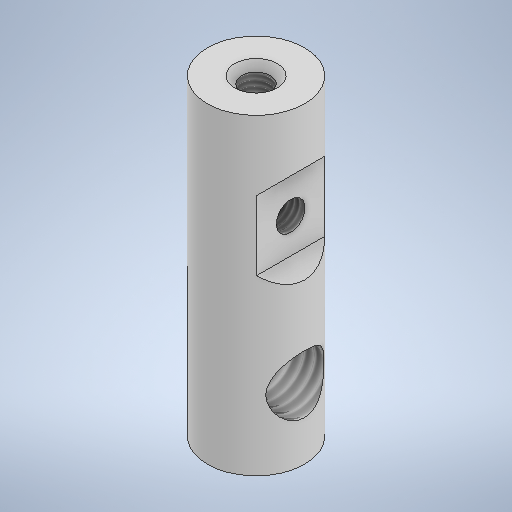
# Autodesk Inventor part: TS_V1_Fallmagazin_Zylinderanbindung_int
Saved by Autodesk Inventor 2025.2 (Build 292293000, 293)
## iProperties
Created: 2025-06-13
Part Number: TS_V1_Fallmagazin_Zylinderanbindung_int
Material: Generisch
Document SubType Name: Modeling
Designer: tino
Density: 1 g/cm^3
Appearance: Vorgabe
Author: tino
Autodesk Inventor part; units mm, degrees
ref_plane "XY Plane" through (0, 0, 0) normal (0, 0, 1) x (1, 0, 0)
sketch "Skizze1" plane through (0, 0, 0) normal (0, 0, 1) x (1, 0, 0)
  circle A0 centre (0, 0) radius 7
  dimension "d0" = 14
  constraints: 1 centre point, 1 coincident
  measures "d0" diameter of A0
extrude "Extrusion1" add sketch "Skizze1" along normal blind 45
sketch "Skizze2" plane through (0, 0, 45) normal (0, 0, 1) x (1, 0, 0)
  circle A0 centre (0, 0) radius 7 projected
hole "Bohrung1" at (0, 0, 45) direction (0, 0, -1) diameter 4.134 depth 11.5 tip angle 118 thread size "M5x0.8" class "6H" standard "ISO Metric profile"
chamfer "Fasen1" distance 1 angle 45 1 edges at (0, 2.067, 45)
ref_plane "Arbeitsebene1" through (-7, 0, 0) normal (1, 0, 0) x (0, 1, 0)
ref_plane "Arbeitsebene2" through (0, -7, 0) normal (0, 1, 0) x (-1, 0, 0)
ref_plane "Arbeitsebene3" through (7, 0, 0) normal (1, 0, 0) x (0, 1, 0)
sketch "Skizze6" plane through (7, 0, 0) normal (1, 0, 0) x (0, 1, 0)
  line L0 (-7, 0) -> (-7, 45) projected
  line L1 (7, 0) -> (7, 45) projected
  line L2 (-7, 25) -> (7, 25)
  line L3 (7, 25) -> (7, 35)
  line L4 (7, 35) -> (-7, 35)
  line L5 (-7, 35) -> (-7, 25)
  line L6 (7, 45) -> (-7, 45) projected
  point P0 (0, 0)
  point P1 (-7, 35)
  dimension "d29" = 10
  dimension "d30" = 10
  constraints: 8 end point, 2 parallel, 2 point on line, 1 horizontal, 1 perpendicular
  measures "d29" distance of L3.end L2.end
  measures "d30" distance between parallel lines of L6 L4
extrude "Extrusion4" cut sketch "Skizze6" against normal blind 2 contours L0 L4 L1 L2
sketch "Skizze7" plane through (5, 0, 0) normal (1, 0, 0) x (0, 0, -1)
  line L0 (-25, -4.899) -> (-25, 4.899) projected
  line L1 (0, 7) -> (0, -7) projected
  point P0 (0, 0)
  point P1 (-30, 0)
  point P2 (0, 0)
  point P3 (0, 0)
  point P4 (0, 0)
  dimension "d33" = 5
  constraints: 1 horizontal alignment, 1 midpoint
  measures "d33" distance from line of point (-30, 0) L0
hole "Bohrung3" at (5, 0, 30) direction (-1, 0, 0) diameter 4.134 end through all thread size "M5x0.8" class "6H" standard "ISO Metric profile"
ref_plane "Arbeitsebene4" through (0, 7, 0) normal (0, 1, 0) x (-1, 0, 0)
sketch "Skizze8" plane through (0, 7, 0) normal (0, 1, 0) x (-1, 0, 0)
  line L0 (-5, 25) -> (-5, 25) projected
  line L1 (-5, 27.933) -> (-5, 32.067) projected
  line L2 (-5, 25) -> (-5, 35) projected
  line L3 (-5, 35) -> (-5, 25) projected
  line L4 (-5, 35) -> (-7, 35) projected
  line L5 (-5, 35) -> (-5, 25) projected
  line L6 (-5, 25) -> (-5, 35) projected
  line L7 (-5, 35) -> (-5, 35) projected
  line L8 (-7, 25) -> (-5, 25) projected
  line L9 (-5, 25) -> (-7, 23)
  line L10 (-7, 0) -> (-7, 45) projected
  line L11 (-5, 25) -> (-2.1716, 25) construction
  line L12 (-7, 23) -> (-7, 25)
  line L13 (-5, 35) -> (-7, 37)
  line L14 (-5, 35) -> (-2.1716, 35) construction
  line L15 (-7, 37) -> (-7, 35)
  point P0 (0, 0)
  point P1 (-5, 24.433)
  point P2 (-5, 28.567)
  dimension "d42" = 135
  dimension "d43" = 135
  constraints: 12 end point, 2 equal length, 2 horizontal, 2 point on line, 1 collinear, 1 perpendicular
  measures "d42" angle of L9 L11
  measures "d43" angle of L14 L13
extrude "Extrusion5" cut sketch "Skizze8" against normal through all contours L9 L10 L8 | L4 L10 L13
sketch "Skizze9" plane through (-7, 0, 0) normal (1, 0, 0) x (0, 1, 0)
  line L0 (7, 0) -> (7, 45) projected
  line L1 (-7, 0) -> (-7, 45) projected
  line L2 (7, 0) -> (-7, 0)
  line L3 (-7, 0) -> (-7, 20)
  line L4 (-7, 20) -> (7, 20)
  line L5 (7, 20) -> (7, 0)
  point P0 (0, 0)
  point P1 (7, 20)
  dimension "d46" = 20
  constraints: 8 end point, 2 parallel, 2 point on line, 1 horizontal, 1 midpoint, 1 perpendicular
  measures "d46" distance between parallel lines of L2 L4
extrude "Extrusion6" cut sketch "Skizze9" along normal blind 2
sketch "Skizze10" plane through (0, -7, 0) normal (0, 1, 0) x (-1, 0, 0)
  line L0 (7, 20) -> (5, 20) projected
  line L1 (5, 20) -> (5, 20) projected
  line L2 (5, 20) -> (7, 22)
  line L3 (7, 20) -> (7, 45) projected
  line L4 (5, 20) -> (7.8284, 20) construction
  point P0 (0, 0)
  dimension "d49" = 45
  constraints: 4 end point, 1 equal length, 1 horizontal, 1 point on line
  measures "d49" angle of L4 L2
extrude "Extrusion7" cut sketch "Skizze10" along normal through all
sketch "Skizze11" plane through (-5, 0, 0) normal (-1, 0, 0) x (0, 0, 1)
  line L0 (0, -4.899) -> (0, 4.899) projected
  point P0 (0, 0)
  point P1 (10, 0)
  point P2 (0, 0)
  point P3 (0, 0)
  dimension "d52" = 10
  constraints: 2 midpoint, 1 horizontal alignment
  measures "d52" distance of point (0, 0) point (10, 0)
hole "Bohrung4" at (-5, 0, 10) direction (1, 0, 0) diameter 8.376 end through all thread size "M10x1.5" class "6H" standard "ISO Metric profile"
